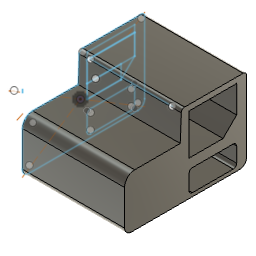
light_robot_containment (Autodesk Fusion 360 design; units mm, degrees)
Autodesk Fusion 360 part; units mm, degrees
sketch "Sketch1" plane through (0, 0, 0) normal (1, 0, 0) x (0, 1, 0)
  line L0 (-75, -56.7965) -> (84.5885, -56.7965)
  line L1 (94.5885, -46.7965) -> (94.5885, 58.2035)
  line L2 (89.5885, 63.2035) -> (3.5272, 63.2035)
  line L3 (-70, 20.0323) -> (-2.9575, 20.0323)
  line L4 (-2.9575, 20.0323) -> (-1.469, 58.3973)
  line L5 (-97.4281, 59.7817) -> (-104.34, 62.6519) construction
  line L6 (-1.3367, 61.8082) -> (1.7233, 63.2035) construction
  line L7 (-85, 23.6607) -> (-92.9575, 20.0323) construction
  line L8 (-85, 51.039) -> (-85, 54.6209)
  line L9 (-85, 5.0323) -> (-85, -46.7965)
  line L10 (94.5885, -56.7965) -> (-33.3617, 20.0323) construction
  line L11 (-104.34, 62.6519) -> (-85, 51.039) construction
  line L12 (79.9542, 44.9695) -> (9.9542, 44.9695)
  line L13 (9.9542, 44.9695) -> (9.9542, 14.9695)
  line L14 (79.9542, 14.9695) -> (79.9542, 44.9695)
  line L15 (9.8967, -5.088) -> (59.8985, -5.088)
  line L16 (9.8971, 14.912) -> (9.8967, -5.088)
  line L17 (67.3, 44.9695) -> (94.5885, 63.2035) construction
  line L18 (79.9542, 14.9695) -> (59.8985, -5.088)
  line L19 (-85, -56.7965) -> (9.8969, 6.6131) construction
  line L20 (22.3522, 14.9356) -> (22.4384, 14.9932) construction
  line L21 (79.9542, 44.9695) -> (9.8971, 44.9695)
  line L22 (9.8971, 44.9695) -> (9.8971, 14.912)
  line L23 (9.8971, 14.912) -> (79.9542, 14.912)
  line L24 (79.9542, 14.912) -> (79.9542, 44.9695)
  line L25 (9.9542, 14.9695) -> (59.8985, 14.9695)
  line L26 (59.8985, 14.9695) -> (59.8985, -5.088)
  line L27 (59.8985, -5.088) -> (9.9542, -5.088)
  line L28 (9.9542, -5.088) -> (9.9542, 14.9695)
  arc A0 (-70, 20.0323) -> (-85, 5.0323) centre (-70, 5.0323) ccw
  arc A1 (84.5885, -56.7965) -> (94.5885, -46.7965) centre (84.5885, -46.7965) ccw
  arc A2 (-85, -46.7965) -> (-75, -56.7965) centre (-75, -46.7965) ccw
  arc A3 (94.5885, 58.2035) -> (89.5885, 63.2035) centre (89.5885, 58.2035) ccw
  arc A4 (3.5272, 63.2035) -> (-1.469, 58.3973) centre (3.5272, 58.2035) ccw
  line L29 (79.9542, 44.9695) -> (9.9542, 44.9695)
  line L30 (9.9542, 44.9695) -> (9.9542, 54.9695)
  line L31 (9.9542, 54.9695) -> (79.9542, 54.9695)
  line L32 (79.9542, 54.9695) -> (79.9542, 44.9695)
  line L33 (74.9542, -19.6144) -> (14.9542, -19.6144)
  line L34 (9.9542, -24.6144) -> (9.9542, -46.6144)
  line L35 (14.9542, -51.6144) -> (74.9542, -51.6144)
  line L36 (79.9542, -46.6144) -> (79.9542, -24.6144)
  arc A5 (14.9542, -19.6144) -> (9.9542, -24.6144) centre (14.9542, -24.6144) ccw
  arc A6 (9.9542, -46.6144) -> (14.9542, -51.6144) centre (14.9542, -46.6144) ccw
  arc A7 (79.9542, -24.6144) -> (74.9542, -19.6144) centre (74.9542, -24.6144) ccw
  arc A8 (74.9542, -51.6144) -> (79.9542, -46.6144) centre (74.9542, -46.6144) ccw
  point P0 (79.9542, -19.6144)
  point P1 (9.9542, -19.6144)
  point P2 (79.9542, -51.6144)
  dimension "d1" = 180
  dimension "d2" = 120
  dimension "d3" = 90
  dimension "d4" = 40
  dimension "d5" = 70
  dimension "d6" = 30
  dimension "d10" = 15
  dimension "d11" = 10
  dimension "d12" = 10
  dimension "d13" = 5
  dimension "d14" = 5
  dimension "d15" = 70
  dimension "d16" = 10
  dimension "d17" = 70
  dimension "d18" = 32
  dimension "d19" = 5
  dimension "d20" = 5
  dimension "d21" = 5
  dimension "d22" = 5
  constraint horizontal L0
  constraint perpendicular L0 L1
  constraint parallel L0 L2
  constraint parallel L1 L8
  constraint coincident origin L19
  constraint coincident origin L10
  constraint coincident L7.start L8
  constraint collinear L6 L7
  constraint coincident L5 L8.end
  constraint collinear L8 L9
  constraint collinear L10 L11
  constraint coincident L3 L10.end
  constraint horizontal L12
  constraint perpendicular L12 L13
  constraint parallel L13 L14
  constraint horizontal L15
  constraint coincident L12 L17.start
  constraint collinear L17 L19
  constraint coincident L16 L19.end
  constraint collinear L19 L20
  constraint horizontal L21
  constraint vertical L22
  constraint horizontal L23
  constraint vertical L24
  constraint horizontal L25
  constraint vertical L26
  constraint horizontal L27
  constraint vertical L28
  constraint coincident L7.end L3
  constraint tangent L3 A0
  constraint tangent L9 A0
  constraint coincident L10.start L1
  constraint coincident L10.start L0
  constraint tangent L1 A1
  constraint tangent L0 A1
  constraint coincident L19.start L9
  constraint coincident L19.start L0
  constraint tangent L9 A2
  constraint tangent L0 A2
  constraint coincident L17.end L2
  constraint coincident L17.end L1
  constraint tangent L2 A3
  constraint tangent L1 A3
  constraint coincident L2 L6.end
  constraint coincident L6.start L4
  constraint tangent L2 A4
  constraint tangent L4 A4
  constraint horizontal L29
  constraint vertical L30
  constraint horizontal L31
  constraint vertical L32
  constraint horizontal L33
  constraint vertical L34
  constraint horizontal L35
  constraint vertical L36
  constraint coincident P1 L33
  constraint coincident P1 L34
  constraint tangent L33 A5
  constraint tangent L34 A5
  constraint tangent L34 A6
  constraint tangent L35 A6
  constraint coincident P0 L33
  constraint coincident P0 L36
  constraint tangent L33 A7
  constraint tangent L36 A7
  constraint coincident P2 L36
  constraint coincident P2 L35
  constraint tangent L36 A8
  constraint tangent L35 A8
  measures "d1" distance of L17.end L8.start
  measures "d2" distance of L10.start L17.end
  measures "d3" distance of L7.end L3.end
  measures "d4" distance of L5.start L7.end
  measures "d5" distance of L13.end L14.start
  measures "d6" distance of L12.end L13.end
  measures "d10" radius of A0
  measures "d11" radius of A1
  measures "d12" radius of A2
  measures "d13" radius of A3
  measures "d14" radius of A4
  measures "d15" distance of L12.start L12.end
  measures "d16" distance of L12.start L31.end
  measures "d17" distance of P0 P1
  measures "d18" distance of P0 P2
  measures "d19" radius of A5
  measures "d20" radius of A6
  measures "d21" radius of A7
  measures "d22" radius of A8
extrude "Extrude1" add sketch "Sketch1" along normal blind 150
sketch "Sketch2" plane through (0, 0, 0) normal (0, 1, 0) x (1, 0, 0)
  line L0 (15.2809, -58.615) -> (135.2809, -58.615)
  constraint horizontal L0
